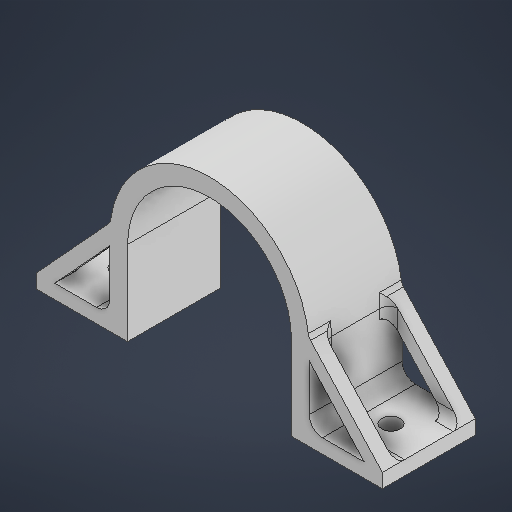
# Autodesk Inventor part: доп крепл мотора 25-26
Saved by Autodesk Inventor 2025 (Build 290162000, 162)
## iProperties
Created: 2025-09-24
Part Number: доп крепл мотора 25-26
Material: Типовые
Document SubType Name: Modeling
Designer: GameHD
Density: 1 g/cm^3
Appearance: По умолчанию
Author: GameHD
Autodesk Inventor part; units mm, degrees
ref_plane "YZ Plane" through (0, 0, 0) normal (1, 0, 0) x (0, 1, 0)
ref_plane "XZ Plane" through (0, 0, 0) normal (0, 1, 0) x (-1, 0, 0)
ref_plane "XY Plane" through (0, 0, 0) normal (0, 0, 1) x (1, 0, 0)
sketch "Эскиз1" plane through (0, 0, 0) normal (0, 0, 1) x (1, 0, 0)
  arc A0 (18.5, 0) -> (-18.5, 0) centre (0, 0) ccw
  line L0 (-22.5, 0) -> (22.5, 0)
  arc A1 (22.5, 0) -> (-22.5, 0) centre (0, 0) ccw
  line L1 (-22.5, 0) -> (-22.5, -12.8)
  line L2 (-22.5, -19) -> (-35.5, -19)
  line L3 (-35.5, -19) -> (-35.5, -15.8)
  line L4 (-35.5, -15.8) -> (-25.5, -15.8)
  arc A2 (-25.5, -15.8) -> (-22.5, -12.8) centre (-25.5, -12.8) ccw
  line L5 (-18.5, 0) -> (-18.5, -19)
  line L6 (-18.5, -19) -> (-22.5, -19)
  line L7 (0, 0) -> (0, 6.7823)
  line L8 (22.5, 0) -> (22.5, -12.8)
  line L9 (22.5, -19) -> (35.5, -19)
  line L10 (35.5, -19) -> (35.5, -15.8)
  line L11 (35.5, -15.8) -> (25.5, -15.8)
  arc A3 (22.5, -12.8) -> (25.5, -15.8) centre (25.5, -12.8) ccw
  line L12 (18.5, 0) -> (18.5, -19)
  line L13 (18.5, -19) -> (22.5, -19)
  dimension "d0" = 37
  dimension "d1" = 45
  dimension "d2" = 13
  dimension "d3" = 3.2
  dimension "d4" = 3
  constraints: 28 end point, 8 point on circle, 8 symmetric about line, 4 centre point, 4 perpendicular, 3 point on line, 3 tangent, 2 coincident, 2 horizontal, 2 vertical, 1 other
  measures "d0" diameter of A0
  measures "d1" diameter of A1
  measures "d2" distance of L2.start L2.end
  measures "d3" distance of L2.end L3.end
  measures "d4" radius of A2
extrude "Выдавливание1" add sketch "Эскиз1" along normal blind 15 contours A0 L0 A1 | L0 L8 A3 L11 L10 L9 L13 L12 | L5 L6 L2 L3 L4 A2 L1 L0
sketch "Эскиз2" plane through (-35.5, -15.8, 0) normal (0, 1, 0) x (1, 0, 0)
  line L0 (71, 0) -> (61, 0) projected
  line L1 (61, 0) -> (61, -15) projected
  line L2 (71, -15) -> (61, -15) projected
  line L3 (71, 0) -> (71, -15) projected
  line L4 (71, -7.5) -> (0, -7.5)
  line L5 (0, 0) -> (0, -15) projected
  line L6 (10, 0) -> (0, 0) projected
  line L7 (10, 0) -> (10, -15) projected
  line L8 (10, -15) -> (0, -15) projected
  line L9 (5, -15) -> (5, 0)
  circle A0 centre (5, -7.5) radius 2.1
  line L10 (35.5, 0) -> (35.5, -25.4)
  circle A1 centre (66, -7.5) radius 2.1
  dimension "d7" = 4.2
  constraints: 6 end point, 5 midpoint, 2 centre point, 1 symmetric about line, 1 vertical, 1 other
  measures "d7" diameter of A0
extrude "Выдавливание2" cut sketch "Эскиз2" against normal blind 20 contours A1 L4 | L4 A1 | A0 L9 L4 | L4 L9 A0 | L9 A0 L4 | L4 A0 L9
sketch "Эскиз3" plane through (0, 0, 15) normal (0, 0, 1) x (1, 0, 0)
  line L0 (35.5, -15.8) -> (39.0359, -15.8)
  line L1 (22.5, 0) -> (37, -15.8)
  line L2 (21.3948, -1.0142) -> (35.8948, -16.8142)
  line L3 (22.3766, 2.3529) -> (39.0359, -15.8)
  line L4 (-18.5, -19) -> (-18.5, 0) projected
  arc A0 (18.5, 0) -> (-18.5, 0) centre (0, 0) ccw projected
  line L5 (18.5, 0) -> (18.5, -19) projected
  line L6 (18.5, -19) -> (35.5, -19) projected
  line L7 (35.5, -19) -> (35.5, -15.8) projected
  line L8 (35.5, -15.8) -> (25.5, -15.8) projected
  arc A1 (22.5, -12.8) -> (25.5, -15.8) centre (25.5, -12.8) ccw projected
  line L9 (22.5, -12.8) -> (22.5, 0) projected
  arc A2 (22.5, 0) -> (-22.5, 0) centre (0, 0) ccw projected
  line L10 (-22.5, 0) -> (-22.5, -12.8) projected
  arc A3 (-25.5, -15.8) -> (-22.5, -12.8) centre (-25.5, -12.8) ccw projected
  line L11 (-25.5, -15.8) -> (-35.5, -15.8) projected
  line L12 (-35.5, -15.8) -> (-35.5, -19) projected
  line L13 (-35.5, -19) -> (-18.5, -19) projected
  line L14 (39.0359, -15.8) -> (35.5, -15.8)
  line L15 (35.5, -15.8) -> (35.5, -19)
  line L16 (35.5, -19) -> (39.0359, -19)
  line L17 (39.0359, -19) -> (39.0359, -15.8)
  line L18 (0, 0) -> (0, 30.1625)
  line L19 (-35.5, -15.8) -> (-39.0359, -15.8)
  line L20 (-22.5, 0) -> (-37, -15.8)
  line L21 (-21.3948, -1.0142) -> (-35.8948, -16.8142)
  line L22 (-22.3766, 2.3529) -> (-39.0359, -15.8)
  line L23 (-18.5, 0) -> (-18.5, -19)
  line L24 (-18.5, -19) -> (-35.5, -19)
  line L25 (-35.5, -19) -> (-35.5, -15.8)
  line L26 (-35.5, -15.8) -> (-25.5, -15.8)
  arc A4 (-25.5, -15.8) -> (-22.5, -12.8) centre (-25.5, -12.8) ccw
  line L27 (-22.5, -12.8) -> (-22.5, 0)
  line L28 (-39.0359, -15.8) -> (-35.5, -15.8)
  line L29 (-35.5, -15.8) -> (-35.5, -19)
  line L30 (-35.5, -19) -> (-39.0359, -19)
  line L31 (-39.0359, -19) -> (-39.0359, -15.8)
  point P0 (22.5, -2.2185)
  point P1 (34.9641, -15.8)
  point P2 (35.5, -16.384)
  point P3 (-34.9641, -15.8)
  point P4 (-22.5, -2.2185)
  dimension "d11" = 1.5
  dimension "d12" = 1.5
  constraints: 44 end point, 12 symmetric about line, 4 parallel, 3 point on circle, 2 horizontal, 2 point on line, 1 centre point, 1 perpendicular, 1 vertical, 1 other
  measures "d11" distance between parallel lines of L1 L2
  measures "d12" distance between parallel lines of L1 L3
extrude "Выдавливание3" add sketch "Эскиз3" along normal blind 3 contours L8 L2 L9 L1 L0 | L0 L17 L16 L7 | L7 L2 L8 | L1 A2 L3 L0 | L7 L6 L5 A0 L18 A2 L9 A1 L8 L2 | L18 A0 L4 L13 L12 L21 L11 A3 L10 A2 | A2 L20 L19 L22 | L10 L21 L11 L19 L20 | L19 L12 L30 L31 | L21 L12 L11
sketch "Эскиз4" plane through (0, 0, 0) normal (0, 0, -1) x (-1, 0, 0)
  line L0 (18.5, -19) -> (18.5, 0) projected
  line L1 (35.5, -19) -> (18.5, -19) projected
  line L2 (35.5, -15.8) -> (35.5, -19) projected
  line L3 (25.5, -15.8) -> (35.5, -15.8) projected
  arc A0 (22.5, -12.8) -> (25.5, -15.8) centre (25.5, -12.8) ccw projected
  line L4 (22.5, 0) -> (22.5, -12.8) projected
  arc A1 (22.5, 0) -> (-22.5, 0) centre (0, 0) ccw projected
  line L5 (-22.5, -12.8) -> (-22.5, 0) projected
  arc A2 (-25.5, -15.8) -> (-22.5, -12.8) centre (-25.5, -12.8) ccw projected
  line L6 (-35.5, -15.8) -> (-25.5, -15.8) projected
  line L7 (-35.5, -19) -> (-35.5, -15.8) projected
  line L8 (-18.5, -19) -> (-35.5, -19) projected
  line L9 (-18.5, 0) -> (-18.5, -19) projected
  arc A3 (18.5, 0) -> (-18.5, 0) centre (0, 0) ccw projected
  line L10 (-35.5, -19) -> (-35.5, -15.8) projected
  line L11 (-35.5, -15.8) -> (-34.9641, -15.8) projected
  line L12 (-22.5, -2.2185) -> (-34.9641, -15.8) projected
  line L13 (-22.5, -2.2185) -> (-22.5, 0) projected
  arc A4 (-22.3766, 2.3529) -> (-22.5, 0) centre (0, 0) ccw projected
  line L14 (-39.0359, -15.8) -> (-22.3766, 2.3529) projected
  line L15 (-39.0359, -19) -> (-39.0359, -15.8) projected
  line L16 (-35.5, -19) -> (-39.0359, -19) projected
  line L17 (35.5, -15.8) -> (35.5, -19) projected
  line L18 (39.0359, -19) -> (35.5, -19) projected
  line L19 (39.0359, -15.8) -> (39.0359, -19) projected
  line L20 (22.3766, 2.3529) -> (39.0359, -15.8) projected
  arc A5 (22.5, 0) -> (22.3766, 2.3529) centre (0, 0) ccw projected
  line L21 (22.5, 0) -> (22.5, -2.2185) projected
  line L22 (34.9641, -15.8) -> (22.5, -2.2185) projected
  line L23 (34.9641, -15.8) -> (35.5, -15.8) projected
  point P0 (-22.3766, 2.3529)
extrude "Выдавливание4" add sketch "Эскиз4" along normal blind 3 contours L0 A3 L9 L8 L7 L6 A2 L5 A1 L4 A0 L3 L2 L1 | L2 L3 L22 L4 A1 L20 L19 L18 | L16 L15 L14 A1 L5 L12 L6 L7
sketch "Эскиз5" plane through (0, 0, 15) normal (0, 0, -1) x (-1, 0, 0)
  line L0 (-35.5, -19) -> (-35.5, -15.8) projected
  line L1 (-35.5, -15.8) -> (-34.9641, -15.8) projected
  line L2 (-22.5, -2.2185) -> (-34.9641, -15.8) projected
  line L3 (-22.5, -2.2185) -> (-22.5, 0) projected
  arc A0 (-22.3766, 2.3529) -> (-22.5, 0) centre (0, 0) ccw projected
  line L4 (-39.0359, -15.8) -> (-22.3766, 2.3529) projected
  line L5 (-39.0359, -19) -> (-39.0359, -15.8) projected
  line L6 (-35.5, -19) -> (-39.0359, -19) projected
  line L7 (35.5, -15.8) -> (35.5, -19) projected
  line L8 (39.0359, -19) -> (35.5, -19) projected
  line L9 (39.0359, -15.8) -> (39.0359, -19) projected
  line L10 (22.3766, 2.3529) -> (39.0359, -15.8) projected
  arc A1 (22.5, 0) -> (22.3766, 2.3529) centre (0, 0) ccw projected
  line L11 (22.5, 0) -> (22.5, -2.2185) projected
  line L12 (34.9641, -15.8) -> (22.5, -2.2185) projected
  line L13 (34.9641, -15.8) -> (35.5, -15.8) projected
  line L14 (39.0359, -15.8) -> (-39.0359, -15.8)
  line L15 (-18.5, -19) -> (-39.0359, -19) projected
  constraints: 2 end point, 1 parallel
extrude "Выдавливание5" add sketch "Эскиз5" along normal up to surface (15 mm away) contours L6 L5 L14 L0 | L14 L9 L8 L7
fillet "Сопряжение1" radius 2 16 edges at (-37, -15.8, 15) (-37, -15.8, 0) (-22.5, -1.1092, 0) (-22.4691, 1.1781, 0) (-22.5, -1.1092, 15) (-22.4691, 1.1781, 15) (22.3766, 2.3529, 16.5) (22.3766, 2.3529, -1.5) (22.5, -1.1092, 0) (22.4691, 1.1781, 0) (37, -15.8, 0) (37, -15.8, 15) (22.4691, 1.1781, 15) (22.5, -1.1092, 15) (-22.3766, 2.3529, 16.5) (-22.3766, 2.3529, -1.5)
